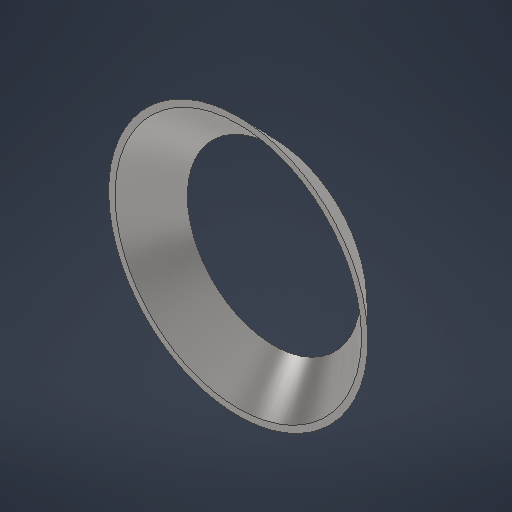
# Autodesk Inventor part: CollegamentoCorpo1
Saved by Autodesk Inventor 2026.2 (Build 302298010, 298A)
## iProperties
Created: 2026-05-01
Part Number: CollegamentoCorpo1
Material: Steel, Alloy
Document SubType Name: Modeling
Designer: Yan
Density: 7.73 g/cm^3
Appearance: Semi-Polished
Author: Yan
Autodesk Inventor part; units mm, degrees
ref_plane "YZ Plane" through (0, 0, 0) normal (1, 0, 0) x (0, 1, 0)
ref_plane "XZ Plane" through (0, 0, 0) normal (0, 1, 0) x (-1, 0, 0)
ref_plane "XY Plane" through (0, 0, 0) normal (0, 0, 1) x (1, 0, 0)
sketch "Sketch1" plane through (0, 0, 0) normal (1, 0, 0) x (0, 1, 0)
  line L0 (0, 0) -> (0, -111)
  line L1 (0, 0) -> (385, 0)
  line L2 (0, -111) -> (270, -111)
  line L3 (270, -111) -> (385, 0)
  line L4 (405, 0) -> (290, -111)
  line L5 (290, -111) -> (270, -111)
  line L6 (405, 0) -> (385, 0)
  dimension "d0" = 20
  dimension "d1" = 385
  dimension "d2" = 270
  dimension "d3" = 111
  constraints: 14 end point, 2 horizontal, 2 parallel, 1 point on line, 1 vertical
  measures "d0" distance of L4.start L1.end
  measures "d1" distance of L0.start L1.end
  measures "d2" distance of L0.end L2.end
  measures "d3" distance of L0.start L0.end
revolve "Revolution1" add sketch "Sketch1" angle 360 about axis through (0, 0, 0) along (0, 0, -1) contours L6 L4 L5 L3
body "Solid1"
